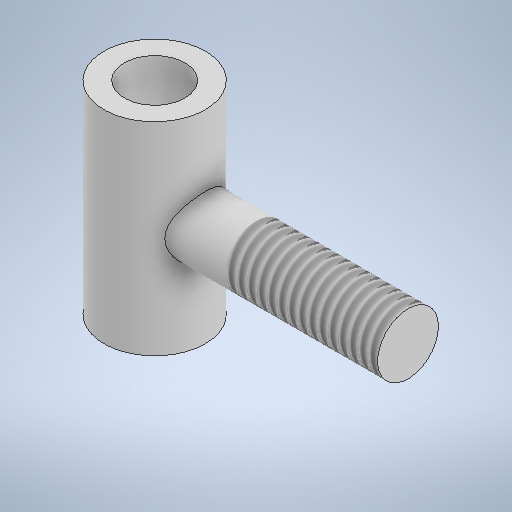
# Autodesk Inventor part: verbindungunten
Saved by Autodesk Inventor 2025.1 (Build 291241000, 241)
## iProperties
Created: 2024-08-07
Part Number: verbindungunten
Material: Generisch
Document SubType Name: Modeling
Designer: ffogue
Density: 1 g/cm^3
Appearance: Vorgabe
Author: ffogue
Autodesk Inventor part; units mm, degrees
ref_plane "XZ Plane" through (0, 0, 0) normal (0, 1, 0) x (-1, 0, 0)
ref_plane "XY Plane" through (0, 0, 0) normal (0, 0, 1) x (1, 0, 0)
sketch "Sketch1" plane through (0, 0, 0) normal (0, 0, 1) x (1, 0, 0)
  circle A0 centre (0, 0) radius 5
  dimension "d0" = 10
  constraints: 1 centre point, 1 coincident
  measures "d0" diameter of A0
extrude "Extrusion1" add sketch "Sketch1" along normal blind 20
sketch "Sketch2" plane through (0, 0, 20) normal (0, 0, 1) x (1, 0, 0)
  circle A0 centre (0, 0) radius 5 projected
  constraints: 1 coincident
hole "Hole1" at (0, 0, 20) direction (0, 0, -1) diameter 6 depth 8
ref_plane "Work Plane1" through (25, 0, 0) normal (1, 0, 0) x (0, 1, 0)
sketch "Sketch3" plane through (25, 0, 0) normal (1, 0, 0) x (0, 1, 0)
  circle A0 centre (0, 10) radius 3
  line L0 (-5, 0) -> (-5, 20) projected
  point P0 (0, 0)
  point P1 (-5, 10)
  dimension "d11" = 6
  constraints: 1 centre point, 1 horizontal alignment, 1 midpoint, 1 vertical alignment
  measures "d11" diameter of A0
extrude "Extrusion2" add sketch "Sketch3" against normal up to surface
thread "Thread1" size "M6x1" class "6g" standard "ISO Metric profile" length 15
body "Solid1"
